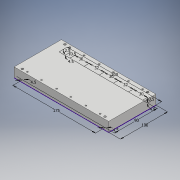
# Autodesk Inventor part: 3lasers1fiberHeatSinkBlock
Saved by Autodesk Inventor 2017 (Build 210142000, 142)
## iProperties
Created: 2017-10-24
Part Number: 3lasers1fiberHeatSinkBlock
Material: Generic
Document SubType Name: Modeling
Designer: nvladim
Density: 1 g/cm^3
Appearance: Default
Author: nvladim
Autodesk Inventor part; units mm, degrees
ref_plane "YZ Plane" through (0, 0, 0) normal (1, 0, 0) x (0, 1, 0)
ref_plane "XZ Plane" through (0, 0, 0) normal (0, 1, 0) x (-1, 0, 0)
ref_plane "XY Plane" through (0, 0, 0) normal (0, 0, 1) x (1, 0, 0)
sketch "Sketch2" plane through (0, 0, 0) normal (0, 0, 1) x (1, 0, 0)
  line L0 (0, 0) -> (200, 0)
  line L1 (200, 0) -> (200, 100)
  line L2 (200, 100) -> (0, 100)
  line L3 (0, 100) -> (0, 0)
  line L4 (0, 5) -> (200, 5) construction
  line L5 (0, 95) -> (200, 95) construction
  circle A0 centre (12.5, 95) radius 2.25
  circle A1 centre (12.5, 5) radius 2.25
  circle A2 centre (187.5, 95) radius 2.25
  circle A3 centre (187.5, 5) radius 2.25
  point P0 (23, 5)
  point P1 (23, 95)
  point P2 (53, 5)
  point P3 (53, 95)
  point P4 (85, 95)
  point P5 (85, 5)
  point P6 (115, 95)
  point P7 (115, 5)
  point P8 (147, 95)
  point P9 (147, 5)
  point P10 (177, 95)
  point P11 (177, 5)
  dimension "d18" = 90
  dimension "d0" = 200
  dimension "d1" = 100
  dimension "d2" = 30
  dimension "d3" = 32
  dimension "d4" = 30
  dimension "d5" = 32
  dimension "d6" = 30
  dimension "d13" = 10.5
  dimension "d15" = 10.5
  dimension "d16" = 12.5
  dimension "d17" = 175
  dimension "d21" = 4.5
  dimension "d22" = 4.5
  dimension "d23" = 4.5
  dimension "d24" = 4.5
  constraints: 8 end point, 6 vertical alignment, 4 centre point, 4 coincident, 4 point on line, 2 parallel, 2 vertical, 1 horizontal, 1 perpendicular, 22 other
  measures "d0" distance of L2.end L1.end
  measures "d1" distance of L1.end L0.end
  measures "d2" distance of point (23, 95) point (53, 95)
  measures "d3" distance of point (85, 95) point (53, 95)
  measures "d4" distance of point (115, 95) point (85, 95)
  measures "d5" distance of point (147, 95) point (115, 95)
  measures "d6" distance of point (177, 95) point (147, 95)
  measures "d13" distance of point (187.5, 95) point (177, 95)
  measures "d15" distance of point (12.5, 95) point (23, 95)
  measures "d16" distance of point (0, 95) point (12.5, 95)
  measures "d17" distance of point (187.5, 5) point (12.5, 5)
  measures "d21" diameter of A0
  measures "d22" diameter of A1
  measures "d23" diameter of A2
  measures "d24" diameter of A3
extrude "Extrusion2" add sketch "Sketch2" along normal blind 20
hole "Hole1" at (23, 5, 0) at (23, 95, 0) at (53, 5, 0) at (53, 95, 0) at (85, 95, 0) at (85, 5, 0) at (115, 95, 0) at (115, 5, 0) at (147, 95, 0) at (147, 5, 0) at (177, 95, 0) at (177, 5, 0) direction (0, 0, 1) diameter 3.242 end through all thread size "M4x0.7" class "6H" standard "ANSI Metric M Profile"
body "Solid2"
